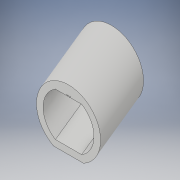
# Autodesk Inventor part: ramp
Saved by Autodesk Inventor 2017 (Build 210142000, 142)
## iProperties
Created: 2018-03-06
Part Number: ramp
Material: Generic
Document SubType Name: Modeling
Designer: braxtonwright
Density: 1 g/cm^3
Appearance: Default
Author: braxtonwright
Autodesk Inventor part; units mm, degrees
ref_plane "YZ Plane" through (0, 0, 0) normal (1, 0, 0) x (0, 1, 0)
ref_plane "XZ Plane" through (0, 0, 0) normal (0, 1, 0) x (-1, 0, 0)
sketch "Sketch1" plane through (0, 0, 0) normal (0, 0, 1) x (1, 0, 0)
  line L0 (-50.8, -84.6667) -> (50.8, -84.6667)
  arc A0 (57.793, -110.0667) -> (-57.793, -110.0667) centre (0, 0) ccw
  arc A1 (-50.8, 84.6667) -> (-50.8, -84.6667) centre (0, 0) ccw
  arc A2 (50.8, -84.6667) -> (50.8, 84.6667) centre (0, 0) ccw
  line L1 (-57.793, -110.0667) -> (57.793, -110.0667)
  line L2 (0, 84.6667) -> (8.9958, 84.6667) construction
  arc A3 (7.4083, 86.2542) -> (8.9958, 84.6667) centre (8.9958, 86.2542) ccw
  arc A4 (-8.9958, 84.6667) -> (-7.4083, 86.2542) centre (-8.9958, 86.2542) ccw
  line L3 (0, 84.6667) -> (0, 87.8417) construction
  line L4 (-7.4083, 87.8417) -> (-7.4083, 86.2542)
  line L5 (7.4083, 87.8417) -> (7.4083, 86.2542)
  line L6 (-7.4083, 87.8417) -> (7.4083, 87.8417)
  line L7 (-8.9958, 84.6667) -> (0, 84.6667) construction
  line L8 (0, 84.646) -> (0, 87.8417) construction
  line L9 (4.1034, 84.646) -> (0, 84.646)
  line L10 (6.35, 87.8417) -> (0, 87.8417)
  line L11 (6.3485, 84.6667) -> (3.1743, 87.8409) construction
  line L12 (6.35, 87.8417) -> (6.35, 86.6178)
  arc A5 (4.1034, 84.646) -> (6.35, 86.6178) centre (4.1034, 86.9117) ccw
  arc A6 (6.35, 87.8417) -> (3.1736, 84.646) centre (6.3485, 84.6667) ccw construction
  line L13 (7.4083, 87.8417) -> (-7.4083, 87.8417)
  line L14 (-4.1034, 84.646) -> (0, 84.646)
  line L15 (-6.35, 87.8417) -> (0, 87.8417)
  line L16 (-6.3485, 84.6667) -> (-3.1743, 87.8409) construction
  line L17 (-6.35, 87.8417) -> (-6.35, 86.6178)
  arc A7 (-6.35, 86.6178) -> (-4.1034, 84.646) centre (-4.1034, 86.9117) ccw
  arc A8 (-3.1736, 84.646) -> (-6.35, 87.8417) centre (-6.3485, 84.6667) ccw construction
  line L18 (-50.8, 84.6667) -> (-8.9958, 84.6667)
  line L19 (8.9958, 84.6667) -> (50.8, 84.6667)
  dimension "d1" = 101.6
  dimension "d2" = 25.4
  dimension "d34" = 14.8167
  dimension "d35" = 1.5875
  dimension "d36" = 1.5875
  dimension "d37" = 6.35
  dimension "d38" = 3.175
  dimension "d39" = 45
  dimension "d40" = 2.2657
  dimension "d41" = 2.2466
  constraints: 40 end point, 20 point on circle, 11 symmetric about line, 9 centre point, 6 horizontal, 4 coincident, 4 point on line, 3 tangent, 2 collinear, 2 midpoint, 2 perpendicular, 2 vertical, 3 other
  measures "d1" distance of L18.start L19.end
  measures "d2" distance between parallel lines of L0 L1
  measures "d34" distance of L4.start L6.end
  measures "d35" distance from line of L2.end L5
  measures "d36" radius of A3
  measures "d37" distance of L15.end L17.start
  measures "d38" distance of L17.start L16.start
  measures "d39" angle of L15 L16
  measures "d40" radius of A7
  measures "d41" horizontal distance of L14.start L17.end
ref_plane "Work Plane2" through (0, 0, 203.2) normal (0, 0, 1) x (1, 0, 0)
sketch "Sketch6" plane through (0, 0, 0) normal (1, 0, 0) x (0, 1, 0)
  line L0 (-110.0667, 0) -> (124.3169, 0) projected
  line L1 (-83.4784, 0) -> (-200.0291, 166.4517)
  point P0 (0, 0)
  dimension "d28" = 203.2
  dimension "d29" = 55
  constraints: 2 end point, 1 point on line
  measures "d28" distance of L1.start L1.end
  measures "d29" angle of L0 L1
sweep "ramp" add profiles "Sketch1" path "Sketch6" path curves L1
sweep "light angle" add profiles "Sketch1" path "Sketch6" separate body path curves L1 contours L6 L12 A5 L9 L14 A7 L17
equation "\"d35\" = 0.5 * d42"
equation "\"d42\" = 3.175"
body "Solid1"
body "Solid2"
